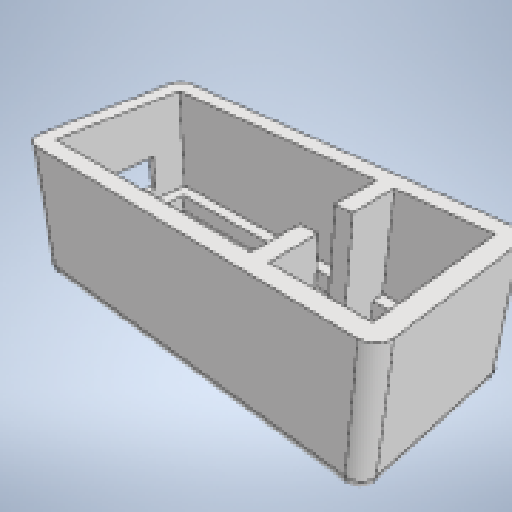
# Autodesk Inventor part: rf_tester_bottom
Saved by Autodesk Inventor 2025 (Build 290162000, 162)
## iProperties
Created: 2025-01-11
Part Number: rf_tester_bottom
Material: Generic
Document SubType Name: Modeling
Designer: Jacob
Density: 1 g/cm^3
Appearance: Default
Author: Jacob
Autodesk Inventor part; units mm, degrees
ref_plane "YZ Plane" through (0, 0, 0) normal (1, 0, 0) x (0, 1, 0)
ref_plane "XZ Plane" through (0, 0, 0) normal (0, 1, 0) x (-1, 0, 0)
ref_plane "XY Plane" through (0, 0, 0) normal (0, 0, 1) x (1, 0, 0)
sketch "Sketch1" plane through (0, 0, 0) normal (0, 1, 0) x (-1, 0, 0)
  line L0 (0, 0) -> (-44.5, 0)
  line L1 (-44.5, 0) -> (-44.5, -18)
  line L2 (-44.5, -18) -> (0, -18)
  line L3 (0, -18) -> (0, 0)
  line L4 (2.4, -20.4) -> (-46.9, -20.4)
  line L5 (-46.9, -20.4) -> (-46.9, 2.4)
  line L6 (-46.9, 2.4) -> (2.4, 2.4)
  line L7 (2.4, 2.4) -> (2.4, -20.4)
  dimension "d0" = 18
  dimension "d1" = 44.5
  dimension "d2" = 2.4
  constraints: 16 end point, 4 parallel, 2 perpendicular, 1 horizontal, 3 other
  measures "d0" distance of L2.end L0.start
  measures "d1" distance of L1.end L2.end
  measures "d2" distance between parallel lines of L2 L4
extrude "Extrusion1" add sketch "Sketch1" against normal blind 2.4 contours L3 L2 L1 L0 | L4 L5 L6 L7
extrude "Extrusion2" add sketch "Sketch1" along normal blind 15.8
sketch "Sketch2" plane through (0, 0, 0) normal (0, 1, 0) x (1, 0, 0)
  line L0 (0, 0) -> (44.5, 0) projected
  line L1 (44.5, 0) -> (44.5, 18) projected
  line L2 (44.5, 18) -> (0, 18) projected
  line L3 (0, 18) -> (0, 0) projected
  line L4 (1.75, 16.25) -> (42.75, 16.25)
  line L5 (42.75, 16.25) -> (42.75, 1.75)
  line L6 (42.75, 1.75) -> (1.75, 1.75)
  line L7 (1.75, 1.75) -> (1.75, 16.25)
  line L8 (32.85, 17.25) -> (42.75, 17.25)
  line L9 (42.75, 17.25) -> (42.75, 0.75)
  line L10 (42.75, 0.75) -> (32.85, 0.75)
  line L11 (32.85, 0.75) -> (32.85, 17.25)
  line L12 (42.75, 13.5) -> (44.5, 13.5)
  line L13 (44.5, 13.5) -> (44.5, 4.5)
  line L14 (44.5, 4.5) -> (42.75, 4.5)
  line L15 (42.75, 4.5) -> (42.75, 13.5)
  line L16 (44.5, 18) -> (44.5, 0) projected
  point P0 (42.75, 9)
  point P1 (44.5, 9)
  point P2 (43.625, 4.5)
  point P3 (42.75, 4.5)
  point P4 (42.75, 13.5)
  dimension "d7" = 1.75
  dimension "d8" = 9.9
  dimension "d9" = 16.5
  dimension "d10" = 9
  constraints: 24 end point, 6 midpoint, 4 parallel, 2 horizontal, 2 perpendicular, 3 other
  measures "d7" distance between parallel lines of L2 L4
  measures "d8" distance of L9.end L10.end
  measures "d9" distance of L8.end L9.end
  measures "d10" distance from line of point (43.625, 4.5) L12
extrude "Extrusion3" add sketch "Sketch2" along normal blind 2.4 contours L3 L2 L1 L12 L5 L9 L8 L11 L4 L7 L6 L10 L14 L0 | L9 L10 L11 L6 | L4 L11 L8 L9
sketch "Sketch3" plane through (0, 2.4, 0) normal (0, 1, 0) x (1, 0, 0)
  line L0 (32.85, 0.75) -> (32.85, 17.25) projected
  line L1 (44.5, 4.5) -> (44.5, 0) projected
  line L2 (44.5, 4.5) -> (42.75, 4.5) projected
  line L3 (42.75, 4.5) -> (42.75, 1.75) projected
  line L4 (42.75, 1.75) -> (1.75, 1.75) projected
  line L5 (1.75, 1.75) -> (1.75, 16.25) projected
  line L6 (1.75, 16.25) -> (42.75, 16.25) projected
  line L7 (42.75, 16.25) -> (42.75, 13.5) projected
  line L8 (42.75, 13.5) -> (44.5, 13.5) projected
  line L9 (44.5, 18) -> (44.5, 13.5) projected
  line L10 (0, 18) -> (44.5, 18) projected
  line L11 (0, 0) -> (0, 18) projected
  line L12 (44.5, 0) -> (0, 0) projected
  line L13 (32.85, 18) -> (30.6, 18)
  line L14 (30.6, 18) -> (30.6, 11.5)
  line L15 (30.6, 11.5) -> (32.85, 11.5)
  line L16 (32.85, 11.5) -> (32.85, 18)
  line L17 (32.85, 0) -> (30.6, 0)
  line L18 (30.6, 0) -> (30.6, 6.5)
  line L19 (30.6, 6.5) -> (32.85, 6.5)
  line L20 (32.85, 6.5) -> (32.85, 0)
  line L21 (44.5, 0) -> (0, 0) projected
  line L22 (0, 18) -> (44.5, 18) projected
  point P0 (30.6, 1.75)
  point P1 (32.85, 1.75)
  point P2 (32.85, 16.25)
  point P3 (30.6, 16.25)
  point P4 (32.85, 0)
  dimension "d13" = 5
  dimension "d14" = 30.6
  constraints: 16 end point, 6 collinear, 4 parallel, 2 horizontal, 2 perpendicular
  measures "d13" distance between parallel lines of L19 L15
  measures "d14" distance between parallel lines of L14 L11
extrude "Extrusion4" add sketch "Sketch3" against normal up to surface (2.4 mm away) contours L0 L4 L18 L19 | L15 L14 L6 L0
extrude "Extrusion5" add sketch "Sketch3" along normal up to surface (13.4 mm away) contours L0 L4 L18 L19 | L15 L14 L6 L0 | L0 L20 L12 L18 L4 | L6 L14 L10 L16 L0
sketch "Sketch4" plane through (0, 2.4, 0) normal (0, 1, 0) x (1, 0, 0)
  line L0 (32.85, 18) -> (32.85, 16.25) projected
  line L1 (32.85, 16.25) -> (42.75, 16.25) projected
  line L2 (42.75, 16.25) -> (42.75, 13.5) projected
  line L3 (42.75, 13.5) -> (44.5, 13.5) projected
  line L4 (44.5, 18) -> (44.5, 13.5) projected
  line L5 (32.85, 18) -> (44.5, 18) projected
  line L6 (32.85, 1.75) -> (32.85, 0) projected
  line L7 (44.5, 0) -> (32.85, 0) projected
  line L8 (44.5, 4.5) -> (44.5, 0) projected
  line L9 (44.5, 4.5) -> (42.75, 4.5) projected
  line L10 (42.75, 4.5) -> (42.75, 1.75) projected
  line L11 (42.75, 1.75) -> (32.85, 1.75) projected
  line L12 (42.75, 16.25) -> (42.75, 18)
  line L13 (42.75, 1.75) -> (42.75, 0)
  point P0 (0, 0)
  constraints: 4 end point, 3 point on line, 1 perpendicular
extrude "Extrusion6" add sketch "Sketch4" along normal blind 4.8 contours L5 L4 L3 L2 L12 | L10 L9 L8 L7 L13
sketch "Sketch5" plane through (-2.4, -2.4, -20.4) normal (-1, 0, 0) x (0, 0, 1)
  line L0 (20.4, 4.8) -> (2.4, 4.8) projected
  line L1 (7.15, 10.9) -> (15.65, 10.9)
  line L2 (15.65, 10.9) -> (15.65, 6.4)
  line L3 (15.65, 6.4) -> (7.15, 6.4)
  line L4 (7.15, 6.4) -> (7.15, 10.9)
  line L5 (11.4, 4.8) -> (11.4, 2.8169) construction
  point P0 (20.4, 2.4)
  point P1 (11.4, 6.4)
  dimension "d21" = 8.5
  dimension "d22" = 4.5
  dimension "d23" = 1.6
  constraints: 10 end point, 2 midpoint, 2 parallel, 1 horizontal, 1 perpendicular, 1 point on line, 1 vertical
  measures "d21" distance of L1.start L1.end
  measures "d22" distance of L3.end L1.start
  measures "d23" distance between parallel lines of L0 L3
extrude "Extrusion7" cut sketch "Sketch5" against normal up to surface (2.4 mm away)
sketch "Sketch6" plane through (-2.4, -2.4, -20.4) normal (-1, 0, 0) x (0, 0, 1)
  line L0 (7.15, 10.9) -> (15.65, 10.9) projected
  line L1 (7.15, 6.4) -> (7.15, 10.9) projected
  line L2 (15.65, 6.4) -> (7.15, 6.4) projected
  line L3 (15.65, 10.9) -> (15.65, 6.4) projected
  line L4 (18.9, 14.15) -> (3.9, 14.15)
  line L5 (3.9, 14.15) -> (3.9, 3.15)
  line L6 (3.9, 3.15) -> (18.9, 3.15)
  line L7 (18.9, 3.15) -> (18.9, 14.15)
  point P0 (20.4, 2.4)
  dimension "d26" = 15
  constraints: 8 end point, 3 other
  measures "d26" distance of L4.start L4.end
extrude "Extrusion8" cut sketch "Sketch6" against normal blind 1.5
fillet "Fillet1" radius 0.5 12 edges at (-1.65, 11.75, -16.5) (-1.65, 11.75, -1.5) (-1.65, 0.75, -1.5) (-1.65, 0.75, -16.5) (-2.4, 11.75, -9) (-2.4, 6.25, -16.5) (-2.4, 0.75, -9) (-2.4, 6.25, -1.5) (-0.9, 0.75, -9) (-0.9, 6.25, -16.5) (-0.9, 11.75, -9) (-0.9, 6.25, -1.5)
fillet "Fillet2" radius 2 8 edges at (22.25, -2.4, -20.4) (-2.4, -2.4, -9) (22.25, -2.4, 2.4) (46.9, -2.4, -9) (46.9, 6.7, 2.4) (46.9, 6.7, -20.4) (-2.4, 6.7, -20.4) (-2.4, 6.7, 2.4)
body "Solid1"
